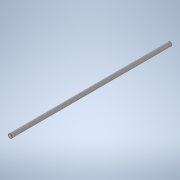
# Autodesk Inventor part: Angle Support
Saved by Autodesk Inventor 2023 (Build 270158000, 158)
## iProperties
Created: 2019-05-30
Part Number: Angle Support
Material: Generic
Document SubType Name: Modeling
Designer: Parker
Density: 1 g/cm^3
Appearance: Default
Author: Parker
Autodesk Inventor part; units mm, degrees
ref_plane "YZ Plane" through (0, 0, 0) normal (1, 0, 0) x (0, 1, 0)
ref_plane "XZ Plane" through (0, 0, 0) normal (0, 1, 0) x (-1, 0, 0)
ref_plane "XY Plane" through (0, 0, 0) normal (0, 0, 1) x (1, 0, 0)
sketch "Sketch1" plane through (0, 0, 0) normal (0, 0, 1) x (1, 0, 0)
  circle A0 centre (0, 0) radius 5
  dimension "d0" = 10
  constraints: 1 centre point, 1 coincident
  measures "d0" diameter of A0
extrude "Extrusion1" add sketch "Sketch1" along normal blind 390
thread "Thread1" size "M10x1.5" class "6g" standard "ANSI Metric M Profile" full length
chamfer "Chamfer1" distance 0.5 angle 45 2 edges at (-5, 0, 390) (-5, 0, 0)
body "Solid1"
